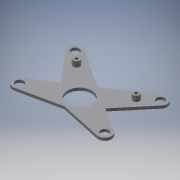
# Autodesk Inventor part: adpaterPlate
Saved by Autodesk Inventor 2017 (Build 210142000, 142)
## iProperties
Created: 2016-11-08
Part Number: adpaterPlate
Material: Generic
Document SubType Name: Modeling
Designer: Camilo
Density: 1 g/cm^3
Appearance: Default
Author: Camilo
Autodesk Inventor part; units mm, degrees
ref_plane "YZ Plane" through (0, 0, 0) normal (1, 0, 0) x (0, 1, 0)
ref_plane "XZ Plane" through (0, 0, 0) normal (0, 1, 0) x (-1, 0, 0)
ref_plane "XY Plane" through (0, 0, 0) normal (0, 0, 1) x (1, 0, 0)
sketch "Sketch1" plane through (0, 0, 0) normal (0, 0, 1) x (1, 0, 0)
  circle A0 centre (0, -7.7) radius 6 construction
  circle A1 centre (18.5, -7.7) radius 2.4 construction
  circle A2 centre (-18.5, -7.7) radius 2.4 construction
  circle A3 centre (0, 12.9) radius 2 construction
  circle A4 centre (-31.7, -20.7) radius 2 construction
  circle A5 centre (31.7, -20.7) radius 2 construction
  circle A6 centre (31.7, 20.7) radius 2 construction
  circle A7 centre (-31.7, 20.7) radius 2 construction
  line L0 (-36.7, -25.7) -> (36.7, -25.7) construction
  line L1 (36.7, -25.7) -> (36.7, 25.7) construction
  line L2 (36.7, 25.7) -> (-36.7, 25.7) construction
  line L3 (-36.7, 25.7) -> (-36.7, -25.7) construction
  circle A8 centre (-31.7, 20.7) radius 3
  circle A9 centre (31.7, 20.7) radius 3
  circle A10 centre (31.7, -20.7) radius 3
  circle A11 centre (-31.7, -20.7) radius 3
  circle A12 centre (-31.7, 20.7) radius 5
  circle A13 centre (31.7, 20.7) radius 5
  circle A14 centre (31.7, -20.7) radius 5
  circle A15 centre (-31.7, -20.7) radius 5
  circle A16 centre (0, -7.7) radius 11
  line L4 (-30.6423, -25.5868) -> (2.3269, -18.4511)
  line L5 (-2.3269, -18.4511) -> (30.6423, -25.5868)
  line L6 (34.378, -16.4776) -> (5.8915, 1.5893)
  line L7 (-34.378, -16.4776) -> (-5.8915, 1.5893)
  line L8 (-28.9219, 24.8572) -> (6.1117, 1.4459)
  line L9 (-35.5281, 17.4835) -> (-8.4217, -14.7764)
  line L10 (-6.1117, 1.4459) -> (28.9219, 24.8572)
  line L11 (35.5281, 17.4835) -> (8.4217, -14.7764)
  circle A17 centre (0, -7.7) radius 9
  point P0 (0, 0)
  dimension "d0" = 1
  dimension "d1" = 2
  dimension "d2" = 5
  dimension "d3" = 3
  constraints: 16 end point, 10 coincident, 9 centre point, 8 point on circle, 8 tangent, 6 equal radius, 18 other
  measures "d0" radial gap between concentric circles of A8 A7
  measures "d1" radial gap between concentric circles of A12 A8
  measures "d3" radial gap between concentric circles of A0 A17
extrude "Extrusion1" add sketch "Sketch1" along normal blind 2
ref_plane "Work Plane1" through (-29.8485, -37.5485, 6) normal (0, 0, 1) x (1, 0, 0)
sketch "Sketch2" plane through (0, 0, 2) normal (0, 0, 1) x (1, 0, 0)
  circle A0 centre (0, -7.7) radius 27.135 construction
  circle A1 centre (31.7, -20.7) radius 3 construction
  line L0 (0, -18.9547) -> (30.6423, -25.5868) construction
  arc A2 (30.6423, -25.5868) -> (34.378, -16.4776) centre (31.7, -20.7) ccw construction
  line L1 (34.378, -16.4776) -> (16.5128, -5.147) construction
  line L2 (16.5128, -5.147) -> (35.5281, 17.4835) construction
  arc A3 (35.5281, 17.4835) -> (28.9219, 24.8572) centre (31.7, 20.7) ccw construction
  line L3 (28.9219, 24.8572) -> (0, 5.53) construction
  line L4 (0, 5.53) -> (-28.9219, 24.8572) construction
  arc A4 (-28.9219, 24.8572) -> (-35.5281, 17.4835) centre (-31.7, 20.7) ccw construction
  line L5 (-35.5281, 17.4835) -> (-16.5128, -5.147) construction
  line L6 (-16.5128, -5.147) -> (-34.378, -16.4776) construction
  arc A5 (-34.378, -16.4776) -> (-30.6423, -25.5868) centre (-31.7, -20.7) ccw construction
  line L7 (-30.6423, -25.5868) -> (0, -18.9547) construction
  circle A6 centre (0, -7.7) radius 9 construction
  circle A7 centre (-31.7, -20.7) radius 3 construction
  circle A8 centre (-31.7, 20.7) radius 3 construction
  circle A9 centre (31.7, 20.7) radius 3 construction
  line L8 (0, -7.7) -> (31.7, 20.7) construction
  line L9 (0, -7.7) -> (-31.7, 20.7) construction
  circle A10 centre (22.2214, 12.2082) radius 2.7 construction
  circle A11 centre (-22.2214, 12.2082) radius 2.7 construction
  circle A12 centre (-22.2214, 12.2082) radius 2.5
  circle A13 centre (22.2214, 12.2082) radius 2.5
  point P0 (0, 0)
  dimension "d7" = 0.2
  dimension "d8" = 5
  constraints: 4 centre point, 4 end point, 2 coincident, 2 equal radius, 2 point on line, 2 tangent
  measures "d7" radial gap between concentric circles of A13 A10
  measures "d8" diameter of A13
extrude "Extrusion2" add sketch "Sketch2" along normal up to surface (4 mm away)
sketch "Sketch3" plane through (-22.2214, 12.2082, 6) normal (0, 0, 1) x (1, 0, 0)
  circle A0 centre (0, 0) radius 1 construction
  circle A1 centre (44.4429, 0) radius 1 construction
  circle A2 centre (0, 0) radius 1.2
  circle A3 centre (44.4429, 0) radius 1.2
  point P0 (22.2214, -12.2082)
  dimension "d11" = 0.2
  constraints: 2 centre point, 2 coincident, 1 equal radius
  measures "d11" radial gap between concentric circles of A0 A2
extrude "Extrusion3" cut sketch "Sketch3" against normal up to surface (4 mm away)
sketch "Sketch5" plane through (0, 0, 2) normal (0, 0, 1) x (1, 0, 0)
  circle A0 centre (-22.2214, 12.2082) radius 2.5 construction
  circle A1 centre (22.2214, 12.2082) radius 2.5 construction
  circle A2 centre (31.7, -20.7) radius 3 construction
  line L0 (0, -18.9547) -> (30.6423, -25.5868) construction
  arc A3 (30.6423, -25.5868) -> (34.378, -16.4776) centre (31.7, -20.7) ccw construction
  line L1 (34.378, -16.4776) -> (16.5128, -5.147) construction
  line L2 (16.5128, -5.147) -> (35.5281, 17.4835) construction
  arc A4 (35.5281, 17.4835) -> (28.9219, 24.8572) centre (31.7, 20.7) ccw construction
  line L3 (28.9219, 24.8572) -> (0, 5.53) construction
  line L4 (0, 5.53) -> (-28.9219, 24.8572) construction
  arc A5 (-28.9219, 24.8572) -> (-35.5281, 17.4835) centre (-31.7, 20.7) ccw construction
  line L5 (-35.5281, 17.4835) -> (-16.5128, -5.147) construction
  line L6 (-16.5128, -5.147) -> (-34.378, -16.4776) construction
  arc A6 (-34.378, -16.4776) -> (-30.6423, -25.5868) centre (-31.7, -20.7) ccw construction
  line L7 (-30.6423, -25.5868) -> (0, -18.9547) construction
  circle A7 centre (0, -7.7) radius 9 construction
  circle A8 centre (-31.7, -20.7) radius 3 construction
  circle A9 centre (-31.7, 20.7) radius 3 construction
  circle A10 centre (31.7, 20.7) radius 3 construction
  line L8 (16.5128, -5.147) -> (-16.5128, -5.147) construction
  line L9 (0, -18.9547) -> (0, 5.53) construction
  line L10 (-25, 9.853) -> (-25, -20.147)
  line L11 (-25, -20.147) -> (25, -20.147)
  line L12 (25, -20.147) -> (25, 9.853)
  line L13 (25, 9.853) -> (-25, 9.853)
  line L14 (-25, 9.853) -> (25, -20.147) construction
  line L15 (-25, -20.147) -> (25, 9.853) construction
  circle A11 centre (0, -7.7) radius 9
  circle A12 centre (0, -7.7) radius 9 projected
  point P0 (0, 0)
  point P1 (0, -5.147)
  dimension "d17" = 30
  dimension "d18" = 50
  constraints: 16 end point, 3 midpoint, 2 horizontal, 2 parallel, 2 perpendicular, 1 centre point, 1 coincident, 1 concentric, 1 point on line
  measures "d17" distance of L10.start L10.end
  measures "d18" distance of L11.end L10.end
extrude "Extrusion5" add sketch "Sketch5" against normal up to surface (2 mm away)
sketch "Sketch4" plane through (0, 0, 2) normal (0, 0, 1) x (1, 0, 0)
  circle A0 centre (-18.5, -7.7) radius 2.4 construction
  circle A1 centre (18.5, -7.7) radius 2.4 construction
  circle A2 centre (18.5, -7.7) radius 2.9
  circle A3 centre (-18.5, -7.7) radius 2.9
  point P0 (0, 0)
  dimension "d14" = 0.5
  constraints: 2 centre point, 2 coincident, 1 equal radius
  measures "d14" radial gap between concentric circles of A2 A1
extrude "Extrusion4" cut sketch "Sketch4" against normal up to surface (2 mm away)
fillet "Fillet1" radius 2 2 edges at (-24.7214, 12.2082, 2) (19.7214, 12.2082, 2)
sketch "Sketch6" plane through (0, 0, 2) normal (0, 0, 1) x (1, 0, 0)
  circle A0 centre (-22.2214, 12.2082) radius 4.5 construction
  circle A1 centre (18.5, -7.7) radius 2.9 construction
  circle A2 centre (-18.5, -7.7) radius 2.9 construction
  circle A3 centre (-31.7, -20.7) radius 3 construction
  circle A4 centre (-31.7, 20.7) radius 3 construction
  circle A5 centre (0, -7.7) radius 9 construction
  circle A6 centre (31.7, 20.7) radius 3 construction
  line L0 (5.5089, -20.147) -> (30.6423, -25.5868) construction
  arc A7 (30.6423, -25.5868) -> (34.378, -16.4776) centre (31.7, -20.7) ccw construction
  line L1 (34.378, -16.4776) -> (25, -10.5299) construction
  line L2 (25, -10.5299) -> (25, 4.9538) construction
  line L3 (25, 4.9538) -> (35.5281, 17.4835) construction
  arc A8 (35.5281, 17.4835) -> (28.9219, 24.8572) centre (31.7, 20.7) ccw construction
  line L4 (28.9219, 24.8572) -> (6.469, 9.853) construction
  line L5 (6.469, 9.853) -> (-6.469, 9.853) construction
  line L6 (-6.469, 9.853) -> (-28.9219, 24.8572) construction
  arc A9 (-28.9219, 24.8572) -> (-35.5281, 17.4835) centre (-31.7, 20.7) ccw construction
  line L7 (-35.5281, 17.4835) -> (-25, 4.9538) construction
  line L8 (-25, 4.9538) -> (-25, -10.5299) construction
  line L9 (-25, -10.5299) -> (-34.378, -16.4776) construction
  arc A10 (-34.378, -16.4776) -> (-30.6423, -25.5868) centre (-31.7, -20.7) ccw construction
  line L10 (-30.6423, -25.5868) -> (-5.5089, -20.147) construction
  line L11 (-5.5089, -20.147) -> (5.5089, -20.147) construction
  circle A11 centre (31.7, -20.7) radius 3 construction
  circle A12 centre (22.2214, 12.2082) radius 4.5 construction
  circle A13 centre (22.2214, 12.2082) radius 1.2 construction
  circle A14 centre (-22.2214, 12.2082) radius 1.2 construction
  arc A15 (-21.7364, 8.7096) -> (21.7364, 8.7096) centre (0, -7.7) ccw construction
  line L12 (21.7364, 8.7096) -> (23.7277, 10.2129) construction
  arc A16 (23.7277, 10.2129) -> (20.4031, 13.9239) centre (22.2214, 12.2082) ccw construction
  line L13 (20.4031, 13.9239) -> (18.6908, 12.1091) construction
  arc A17 (18.6908, 12.1091) -> (-18.6908, 12.1091) centre (0, -7.7) ccw construction
  line L14 (-18.6908, 12.1091) -> (-20.4031, 13.9239) construction
  arc A18 (-20.4031, 13.9239) -> (-23.7277, 10.2129) centre (-22.2214, 12.2082) ccw construction
  line L15 (-23.7277, 10.2129) -> (-21.7364, 8.7096) construction
  circle A19 centre (0, -7.7) radius 25.235 construction
  line L16 (0, -7.7) -> (31.7, -20.7) construction
  line L17 (0, -7.7) -> (-31.7, -20.7) construction
  circle A20 centre (23.348, -17.2749) radius 2.5
  circle A21 centre (-23.348, -17.2749) radius 2.5
  circle A22 centre (22.2214, 12.2082) radius 2.5 projected
  point P0 (0, 0)
  constraints: 4 end point, 2 centre point, 2 equal radius, 2 point on circle, 2 point on line
ref_plane "Work Plane2" through (-27.235, -34.935, 21) normal (0, 0, 1) x (1, 0, 0)
extrude "Extrusion6" add sketch "Sketch6" along normal up to surface (4 mm away) contours A20 | A21
body "Solid1"
